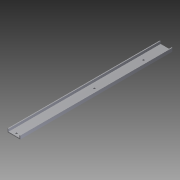
# Autodesk Inventor part: 1
Saved by Autodesk Inventor 2011 (Build 150239000, 239)
## iProperties
Created: 2011-09-24
Part Number: 1
Document SubType Name: Modeling
Designer: Matthew
Density: 1 g/cm^3
Author: Matthew
Autodesk Inventor part; units mm, degrees
ref_plane "YZ Plane" through (0, 0, 0) normal (1, 0, 0) x (0, 1, 0)
ref_plane "XZ Plane" through (0, 0, 0) normal (0, 1, 0) x (-1, 0, 0)
ref_plane "XY Plane" through (0, 0, 0) normal (0, 0, 1) x (1, 0, 0)
sketch "Sketch1" plane through (0, 0, 0) normal (0, 0, 1) x (1, 0, 0)
  line L0 (-11.5809, 11.3971) -> (-46.8809, 11.3971)
  line L1 (-46.8809, 11.3971) -> (-46.8809, 1.8971)
  line L2 (-46.8809, 1.8971) -> (-11.5809, 1.8971)
  line L3 (-11.5809, 1.8971) -> (-11.5809, 11.3971)
  line L4 (-46.8809, 6.6471) -> (-11.5809, 6.6471)
  line L5 (-11.5809, 6.6471) -> (-11.5809, 1.8971)
  line L6 (-11.5809, 4.2721) -> (-46.8809, 4.2721)
  line L7 (-46.8809, 4.2721) -> (-44.5059, 1.8971)
  line L8 (-46.8809, 4.2721) -> (-43.5221, 4.2721) construction
  line L9 (-44.5059, 1.8971) -> (-44.5059, 11.3971)
  line L10 (-11.5809, 4.2721) -> (-13.9559, 1.8971)
  line L11 (-13.9559, 11.3971) -> (-13.9559, 1.8971)
  point P0 (0, 0)
  dimension "d0" = 35.3
  dimension "d1" = 9.5
  dimension "d2" = 45
  constraints: 24 end point, 6 perpendicular, 5 point on line, 3 midpoint, 2 horizontal, 2 parallel, 1 equal length
  measures "d0" distance of L2.end L1.end
  measures "d1" distance of L1.end L0.end
  measures "d2" angle of L7 L8
extrude "Extrusion1" add sketch "Sketch1" along normal blind 450 contours L3 L4 L11 L0 | L3 L6 L11 L4 | L9 L4 L1 L0 | L10 L11 L6 | L3 L2 L10 | L9 L6 L1 L4 | L11 L2 L9 L6 | L9 L7 L6 | L2 L1 L7
sketch "Sketch2" plane through (-44.5059, 4.2721, 0) normal (0, 1, 0) x (1, 0, 0)
  line L0 (30.55, 0) -> (0, 0) projected
  line L1 (0, -450) -> (30.55, -450) projected
  line L2 (15.275, 0) -> (15.275, -26)
  circle A0 centre (15.275, -26) radius 2.15
  line L3 (15.275, -26) -> (15.275, -410)
  line L4 (15.275, -26) -> (15.275, -378)
  circle A1 centre (15.275, -378) radius 2.15
  circle A2 centre (15.275, -410) radius 2.15
  point P0 (44.5059, 0)
  dimension "d5" = 26
  dimension "d6" = 4.3
  dimension "d7" = 384
  dimension "d8" = 352
  constraints: 6 end point, 3 centre point, 3 coincident, 1 collinear, 1 midpoint, 1 perpendicular, 1 point on line
  measures "d5" distance of L2.start L2.end
  measures "d6" diameter of A0
  measures "d7" distance of L3.start L3.end
  measures "d8" distance of L3.start L4.end
extrude "Extrusion2" cut sketch "Sketch2" against normal blind 450
sketch "Sketch3" plane through (0, 0, 450) normal (0, 0, 1) x (1, 0, 0)
  line L0 (-11.5809, 1.8971) -> (-46.8809, 1.8971) projected
  line L1 (-11.5809, 11.3971) -> (-11.5809, 1.8971) projected
  line L2 (-13.9559, 11.3971) -> (-11.5809, 11.3971) projected
  line L3 (-13.9559, 4.2721) -> (-13.9559, 11.3971) projected
  line L4 (-44.5059, 4.2721) -> (-13.9559, 4.2721) projected
  line L5 (-44.5059, 11.3971) -> (-44.5059, 4.2721) projected
  line L6 (-46.8809, 11.3971) -> (-44.5059, 11.3971) projected
  line L7 (-46.8809, 1.8971) -> (-46.8809, 11.3971) projected
  point P0 (0, 0)
extrude "Extrusion3" cut sketch "Sketch3" against normal blind 419.1
sketch "Sketch4" plane through (0, 0, 0) normal (0, 0, -1) x (-1, 0, 0)
  line L0 (11.5809, 1.8971) -> (11.5809, 11.3971) projected
  line L1 (46.8809, 1.8971) -> (11.5809, 1.8971) projected
  line L2 (46.8809, 11.3971) -> (46.8809, 1.8971) projected
  line L3 (44.5059, 11.3971) -> (46.8809, 11.3971) projected
  line L4 (44.5059, 4.2721) -> (44.5059, 11.3971) projected
  line L5 (13.9559, 4.2721) -> (44.5059, 4.2721) projected
  line L6 (13.9559, 11.3971) -> (13.9559, 4.2721) projected
  line L7 (11.5809, 11.3971) -> (13.9559, 11.3971) projected
  point P0 (0, 0)
extrude "Extrusion4" add sketch "Sketch4" against normal blind 426.2437
sketch "Sketch5" plane through (-44.5059, 4.2721, 0) normal (0, 1, 0) x (1, 0, 0)
  line L0 (30.55, 0) -> (0, 0) projected
  line L1 (0, -426.2437) -> (30.55, -426.2437) projected
  line L2 (15.275, 0) -> (15.275, -63.246)
  circle A0 centre (15.275, -63.246) radius 2.3495
  line L3 (15.275, 0) -> (15.275, -203.2)
  line L4 (15.275, -203.2) -> (15.275, -200.8505)
  circle A1 centre (15.275, -200.8505) radius 2.3495
  line L5 (15.275, 0) -> (15.275, -419.1)
  circle A2 centre (15.275, -419.1) radius 2.3495
  point P0 (44.5059, 0)
  dimension "d15" = 63.246
  dimension "d16" = 4.699
  dimension "d17" = 203.2
  dimension "d18" = 2.3495
  dimension "d19" = 419.1
  constraints: 8 end point, 3 coincident, 2 centre point, 2 point on line, 1 collinear, 1 midpoint, 1 perpendicular, 1 vertical alignment, 2 other
  measures "d15" distance of L2.start L2.end
  measures "d16" diameter of A0
  measures "d17" distance of L2.start L3.end
  measures "d18" distance of L3.end L4.end
  measures "d19" distance of L2.start L5.end
extrude "Extrusion5" cut sketch "Sketch5" against normal blind 426.2437
body "Solid1"
